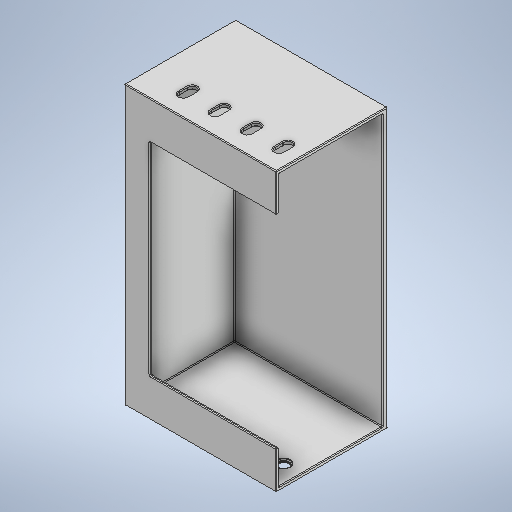
# Autodesk Inventor part: Intake_I2D_Bottom
Saved by Autodesk Inventor 2025 (Build 290162010, 162A)
## iProperties
Created: 2024-10-13
Part Number: Intake_I2D_Bottom
Material: Generic
Document SubType Name: Modeling
Designer: dcfam
Density: 1 g/cm^3
Appearance: Default
Author: dcfam
Autodesk Inventor part; units mm, degrees
ref_plane "YZ Plane" through (0, 0, 0) normal (1, 0, 0) x (0, 1, 0)
ref_plane "XZ Plane" through (0, 0, 0) normal (0, 1, 0) x (-1, 0, 0)
ref_plane "XY Plane" through (0, 0, 0) normal (0, 0, 1) x (1, 0, 0)
sketch "Sketch1" plane through (0, 0, 0) normal (0, 0, 1) x (1, 0, 0)
  line L0 (-30, -55) -> (30, -55)
  line L1 (30, -55) -> (30, 55)
  line L2 (30, 55) -> (-30, 55)
  line L3 (-30, 55) -> (-30, -55)
  line L4 (-30, -55) -> (30, 55) construction
  line L5 (30, -55) -> (-30, 55) construction
  point P0 (0, 0)
  dimension "d0" = 60
  dimension "d1" = 110
  constraints: 12 end point, 2 midpoint, 2 parallel, 1 horizontal, 1 perpendicular
  measures "d0" distance of L2.end L1.end
  measures "d1" distance of L1.end L0.end
extrude "Extrusion1" add sketch "Sketch1" along normal blind 2
sketch "Sketch2" plane through (0, 0, 2) normal (0, 0, 1) x (1, 0, 0)
  line L0 (30, -55) -> (30, 55) projected
  line L1 (30, 55) -> (-30, 55) projected
  line L2 (-30, 55) -> (-30, -55) projected
  line L3 (-30, -55) -> (30, -55) projected
  line L4 (28.5, 53.5) -> (-28.5, 53.5)
  line L5 (-28.5, 53.5) -> (-28.5, -53.5)
  line L6 (-28.5, -53.5) -> (28.5, -53.5)
  line L7 (28.5, -53.5) -> (30, -53.5)
  line L8 (30, -55) -> (30, 55) projected
  line L9 (30, -53.5) -> (30, -55)
  line L10 (28.5, 53.5) -> (30, 53.5)
  line L11 (30, 53.5) -> (30, 55)
  line L12 (30, 55) -> (-30, 55)
  line L13 (-30, 55) -> (-30, -55)
  line L14 (-30, -55) -> (30, -55)
  point P0 (0, 0)
  dimension "d4" = 1.5
  constraints: 20 end point, 4 perpendicular, 2 collinear, 2 point on line, 1 horizontal, 2 other
  measures "d4" distance between parallel lines of L3 L6
extrude "Extrusion2" add sketch "Sketch2" along normal blind 42 contours L3 L2 L1 L0 L10 L4 L5 L6 L7
sketch "Sketch3" plane through (0, 0, 44) normal (0, 0, 1) x (1, 0, 0)
  line L0 (-30, -55) -> (30, -55) projected
  line L1 (30, 55) -> (-30, 55) projected
  line L2 (-30, -55) -> (30, -55)
  line L3 (30, -55) -> (30, 55)
  line L4 (30, 55) -> (-30, 55)
  line L5 (-30, 55) -> (-30, -55)
  point P0 (0, 0)
  constraints: 8 end point, 2 parallel, 1 horizontal, 1 perpendicular
extrude "Extrusion3" add sketch "Sketch3" against normal blind 1
sketch "Sketch4" plane through (0, 0, 44) normal (0, 0, 1) x (1, 0, 0)
  line L0 (20, -40) -> (-20, -40)
  line L1 (-20, -40) -> (-20, 40)
  line L2 (-20, 40) -> (20, 40)
  line L3 (20, -40) -> (-20, 40) construction
  line L4 (-20, -40) -> (20, 40) construction
  line L5 (20, -40) -> (30, -40)
  line L6 (30, 53.5) -> (30, -53.5) projected
  line L7 (20, 40) -> (30, 40)
  line L8 (30, 40) -> (30, -40)
  line L9 (30, -40) -> (30, 40)
  point P0 (0, 0)
  dimension "d9" = 40
  dimension "d10" = 80
  constraints: 18 end point, 3 horizontal, 2 midpoint, 2 perpendicular, 1 collinear, 1 parallel, 1 point on line
  measures "d9" distance of L1.end L2.end
  measures "d10" distance of L0.end L1.end
extrude "Extrusion4" cut sketch "Sketch4" against normal blind 10.525
sketch "Sketch5" plane through (-30, 55, 0) normal (0, 1, 0) x (1, 0, 0)
  arc A0 (54.7, -32.6288) -> (51.3, -32.6288) centre (53, -32.4292) ccw
  line L0 (51.3, -32.6288) -> (51.3, -35.7388)
  line L1 (51.3, -35.7388) -> (51.3, -32.6288)
  line L2 (51.3, -34.1838) -> (58.0274, -34.1838) construction
  arc A1 (51.3, -35.7388) -> (54.7, -35.7388) centre (53, -35.9383) ccw
  line L3 (53, -35.9383) -> (53, -32.4292) construction
  line L4 (54.7, -32.6288) -> (54.7, -35.7388)
  line L5 (60, 0) -> (60, -44) construction
  line L6 (60, 0) -> (0, 0) construction
  line L7 (0, 0) -> (0, -44) construction
  line L8 (60, -44) -> (0, -44) construction
  arc A2 (38.7, -35.7388) -> (42.1, -35.7388) centre (40.4, -35.9383) ccw
  line L9 (42.1, -32.6288) -> (42.1, -35.7388)
  arc A3 (42.1, -32.6288) -> (38.7, -32.6288) centre (40.4, -32.4292) ccw
  line L10 (38.7, -32.6288) -> (38.7, -35.7388)
  arc A4 (26.1, -35.7388) -> (29.5, -35.7388) centre (27.8, -35.9383) ccw
  line L11 (29.5, -32.6288) -> (29.5, -35.7388)
  arc A5 (29.5, -32.6288) -> (26.1, -32.6288) centre (27.8, -32.4292) ccw
  line L12 (26.1, -32.6288) -> (26.1, -35.7388)
  arc A6 (13.5, -35.7388) -> (16.9, -35.7388) centre (15.2, -35.9383) ccw
  line L13 (16.9, -32.6288) -> (16.9, -35.7388)
  arc A7 (16.9, -32.6288) -> (13.5, -32.6288) centre (15.2, -32.4292) ccw
  line L14 (13.5, -32.6288) -> (13.5, -35.7388)
  line L15 (53, -37.65) -> (15.2, -37.65) construction
  line L16 (34.1, -37.65) -> (34.1, -50.35) construction
  point P0 (30, 0)
  point P1 (16.9, -32.6288)
  point P2 (13.5, -35.7388)
  point P3 (16.9, -35.7388)
  point P4 (29.5, -32.6288)
  point P5 (26.1, -35.7388)
  point P6 (29.5, -35.7388)
  point P7 (42.1, -32.6288)
  point P8 (38.7, -35.7388)
  point P9 (42.1, -35.7388)
  point P10 (54.7, -32.6288)
  point P11 (51.3, -35.7388)
  point P12 (54.7, -35.7388)
  dimension "d13" = 3.4
  dimension "d14" = 1.7117
  dimension "d15" = 3.11
  dimension "d16" = 3.11
  dimension "d19" = 12.6
  dimension "d24" = 6.35
  dimension "d37" = 12.7
  dimension "d47" = 32.6288
  dimension "d48" = 1.9726
  dimension "d49" = 1.9726
  dimension "d50" = 35.7388
  dimension "d51" = 1.9726
  dimension "d52" = 35.7388
  dimension "d53" = 5.3726
  dimension "d54" = 32.6288
  dimension "d55" = 14.5726
  dimension "d56" = 35.7388
  dimension "d57" = 14.5726
  dimension "d58" = 35.7388
  dimension "d59" = 17.9726
  dimension "d60" = 32.6288
  dimension "d61" = 27.1726
  dimension "d62" = 35.7388
  dimension "d63" = 27.1726
  dimension "d64" = 35.7388
  dimension "d65" = 30.5726
  dimension "d66" = 32.6288
  dimension "d67" = 39.7726
  dimension "d68" = 35.7388
  dimension "d69" = 39.7726
  dimension "d70" = 35.7388
  dimension "d71" = 43.1726
  dimension "d84" = 5.3
  constraints: 26 end point, 18 point on circle, 8 centre point, 5 symmetric about line, 4 point on line, 3 vertical, 2 horizontal, 2 midpoint, 1 coincident, 1 tangent, 43 other
  measures "d13" distance of A0.start L0.start
  measures "d14" radius of A0
  measures "d15" distance of L0.start L0.end
  measures "d16" distance of L0.end L1.end
  measures "d19" distance of L3.start A2.centre
  measures "d24" distance from line of L8 L15.start
  measures "d37" distance of L16.start L16.end
  measures "d47" distance from line of point (54.7, -32.629) L6
  measures "d49" distance from line of L2.end L5
  measures "d50" distance from line of point (54.7, -35.739) L6
  measures "d52" distance from line of point (51.3, -35.739) L6
  measures "d54" distance from line of point (42.1, -32.629) L6
  measures "d56" distance from line of point (42.1, -35.739) L6
  measures "d58" distance from line of point (38.7, -35.739) L6
  measures "d60" distance from line of point (29.5, -32.629) L6
  measures "d62" distance from line of point (29.5, -35.739) L6
  measures "d64" distance from line of point (26.1, -35.739) L6
  measures "d66" distance from line of point (16.9, -32.629) L6
  measures "d68" distance from line of point (16.9, -35.739) L6
  measures "d70" distance from line of point (13.5, -35.739) L6
  measures "d84" distance between parallel lines of L5 L4
extrude "Extrusion5" cut sketch "Sketch5" against normal blind 25.4
sketch "Sketch6" plane through (-30, -55, 0) normal (0, -1, 0) x (1, 0, 0)
  circle A0 centre (52.992, 34) radius 1.9625
  line L0 (0, 0) -> (0, 44) projected
  line L1 (0, 0) -> (60, 0) projected
  line L2 (60, 0) -> (60, 44) projected
  line L3 (0, 44) -> (60, 44) projected
  circle A1 centre (44.991, 34) radius 1.9625
  circle A2 centre (36.99, 34) radius 1.9625
  circle A3 centre (28.989, 34) radius 1.9625
  line L4 (28.989, 35.9625) -> (52.992, 35.9625) construction
  line L5 (40.9905, 35.9625) -> (40.9905, 52.0375) construction
  point P0 (30, 0)
  dimension "d27" = 3.925
  dimension "d30" = 8.001
  dimension "d35" = 8.0375
  dimension "d36" = 16.075
  dimension "d87" = 7.008
  constraints: 4 end point, 2 centre point, 2 horizontal, 2 vertical alignment, 1 coincident, 1 midpoint, 1 vertical, 10 other
  measures "d30" distance of point (52.992, 34) A1.centre
  measures "d35" distance between parallel lines of L3 L4
  measures "d36" distance of L5.start L5.end
  measures "d87" distance from line of L2 point (52.992, 34)
extrude "Extrusion6" cut sketch "Sketch6" against normal blind 25.4 contours A0 | A1 | A2 | A3
chamfer "Chamfer1" distance 0.5 angle 45 8 edges at (21.0295, -53.5, 34) (13.0285, -53.5, 34) (5.0275, -53.5, 34) (-2.9735, -53.5, 34) (-2.9735, -55, 34) (5.0275, -55, 34) (13.0285, -55, 34) (21.0295, -55, 34)
fillet "Fillet1" radius 0.3 100 edges at (0, -55, 44) (13.0285, -54, 34) (12.5285, -53.5, 34) (21.0295, -54.5, 34) (21.0295, -54, 34) (20.5295, -55, 34) (4.5275, -55, 34) (20.5295, -53.5, 34) (4.5275, -53.5, 34) (-2.9735, -54.5, 34) (-2.9735, -54, 34) (-3.4735, -55, 34) (-3.4735, -53.5, 34) (30, -53.5, 22.5) (30, -55, 22) (0.75, -53.5, 43) (0.75, -53.5, 2) (0, -55, 0) (-28.5, -53.5, 22.5) (-30, -55, 22) (5.0275, -54.5, 34) (13.0285, -54.5, 34) (12.5285, -55, 34) (5.0275, -54, 34) (-20, 0, 43) (-20, 0, 44) (-28.5, 0, 43) (-30, 0, 44) (-30, 0, 0) (0.75, 53.5, 43) (0.75, 53.5, 2) (-28.5, 53.5, 22.5) (0, 55, 44) (0, 55, 0) (-30, 55, 22) (30, 53.5, 22.5) (30, 47.5, 44) (30, 55, 22) (30, 46.75, 43) (30, 0, 0) (30, 0, 2) (30, -47.5, 44) (5, -40, 44) (30, -46.75, 43) (5, -40, 43) (30, -40, 43.5) (-20, -40, 43.5) (-28.5, 0, 2) (30, 40, 43.5) (-20, 40, 43.5) (5, 40, 44) (5, 40, 43) (24.7, 55, 34.1838) (21.3, 53.5, 34.1838) (24.7, 53.5, 34.1838) (23, 53.5, 30.7175) (23, 53.5, 37.65) (21.3, 55, 34.1838) (21.3, 54.25, 32.6288) (23, 55, 30.7175) (24.7, 54.25, 32.6288) (24.7, 54.25, 35.7388) (23, 55, 37.65) (21.3, 54.25, 35.7388) (-13.1, 55, 34.1838) (-13.1, 53.5, 34.1838) (-16.5, 53.5, 34.1838) (-14.8, 53.5, 30.7175) (-13.1, 54.25, 35.7388) (-13.1, 54.25, 32.6288) (-14.8, 55, 30.7175) (-16.5, 55, 34.1838) (-16.5, 54.25, 32.6288) (-16.5, 54.25, 35.7388) (-14.8, 55, 37.65) (-14.8, 53.5, 37.65) (12.1, 53.5, 34.1838) (10.4, 53.5, 37.65) (8.7, 53.5, 34.1838) (10.4, 53.5, 30.7175) (10.4, 55, 30.7175) (10.4, 55, 37.65) (8.7, 54.25, 35.7388) (8.7, 55, 34.1838) (8.7, 54.25, 32.6288) (12.1, 55, 34.1838) (12.1, 54.25, 32.6288) (12.1, 54.25, 35.7388) (-3.9, 53.5, 34.1838) (-2.2, 53.5, 30.7175) (-0.5, 53.5, 34.1838) (-0.5, 54.25, 35.7388) (-0.5, 54.25, 32.6288) (-2.2, 55, 30.7175) (-3.9, 54.25, 35.7388) (-3.9, 54.25, 32.6288) (-3.9, 55, 34.1838) (-2.2, 55, 37.65) (-0.5, 55, 34.1838) (-2.2, 53.5, 37.65)
body "Solid1"
